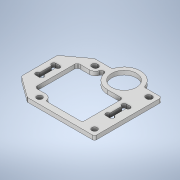
# Autodesk Inventor part: Trunk_chest_side_frame
Saved by Autodesk Inventor 2020.4 (Build 244396000, 396)
## iProperties
Created: 2021-09-08
Part Number: Trunk_chest_side_frame
Material: アルミニウム 2014-T4
Document SubType Name: Modeling
Designer: Masato Kubotera
Density: 2.8 g/cm^3
Appearance: 滑らか - 淡い灰色
Mass: 2.76884 g
Surface Area: 18.8552 cm^2
Volume: 0.988872 cm^3
Description: A2017 T2
Author: moonk
Autodesk Inventor part; units mm, degrees
ref_plane "YZ Plane" through (0, 0, 0) normal (1, 0, 0) x (0, 1, 0)
ref_plane "XZ Plane" through (0, 0, 0) normal (0, 1, 0) x (-1, 0, 0)
ref_plane "XY Plane" through (0, 0, 0) normal (0, 0, 1) x (1, 0, 0)
sketch "スケッチ1" plane through (0, 0, 0) normal (0, 0, 1) x (1, 0, 0)
  circle A0 centre (0, 0) radius 6.05
  arc A1 (2, -7.7976) -> (2, 7.7976) centre (0, 0) ccw
  line L0 (-31, 0) -> (0, 0) construction
  line L1 (-19.51, 24.01) -> (-9.49, 24.01)
  line L2 (-9.49, 24.01) -> (-9.49, 21.99)
  line L3 (-9.49, 21.99) -> (-19.51, 21.99)
  line L4 (-19.51, 21.99) -> (-19.51, 24.01)
  line L5 (-19.51, 24.01) -> (-9.49, 21.99) construction
  line L6 (-9.49, 24.01) -> (-19.51, 21.99) construction
  line L7 (-19.5, 24) -> (-9.5, 24) construction
  line L8 (-9.5, 24) -> (-9.5, 22) construction
  line L9 (-9.5, 22) -> (-19.5, 22) construction
  line L10 (-19.5, 22) -> (-19.5, 24) construction
  line L11 (-19.5, 24) -> (-9.5, 22) construction
  line L12 (-9.5, 24) -> (-19.5, 22) construction
  line L13 (-19.51, 23) -> (-9.49, 23) construction
  arc A2 (-17.41, 24.01) -> (-19.51, 24.01) centre (-18.46, 24.01) ccw
  arc A3 (-19.51, 21.99) -> (-17.41, 21.99) centre (-18.46, 21.99) ccw
  line L14 (-14.5, 24) -> (-14.5, 21.99) construction
  arc A4 (-9.49, 24.01) -> (-11.59, 24.01) centre (-10.54, 24.01) ccw
  arc A5 (-11.59, 21.99) -> (-9.49, 21.99) centre (-10.54, 21.99) ccw
  line L15 (-28, 13.5) -> (-1, 13.5) construction
  line L16 (-1, 13.5) -> (-1, -13.5) construction
  line L17 (-1, -13.5) -> (-28, -13.5) construction
  line L18 (-28, -13.5) -> (-28, 13.5) construction
  line L19 (-28, 13.5) -> (-1, -13.5) construction
  line L20 (-1, 13.5) -> (-28, -13.5) construction
  line L21 (-14.5, 13.5) -> (-14.5, -13.5) construction
  line L22 (-19.51, -10.49) -> (-9.49, -10.49)
  line L23 (-9.49, -10.49) -> (-9.49, -12.51)
  line L24 (-9.49, -12.51) -> (-19.51, -12.51)
  line L25 (-19.51, -12.51) -> (-19.51, -10.49)
  line L26 (-19.51, -10.49) -> (-9.49, -12.51) construction
  line L27 (-9.49, -10.49) -> (-19.51, -12.51) construction
  line L28 (-19.5, -10.5) -> (-9.5, -10.5) construction
  line L29 (-9.5, -10.5) -> (-9.5, -12.5) construction
  line L30 (-9.5, -12.5) -> (-19.5, -12.5) construction
  line L31 (-19.5, -12.5) -> (-19.5, -10.5) construction
  line L32 (-19.5, -10.5) -> (-9.5, -12.5) construction
  line L33 (-9.5, -10.5) -> (-19.5, -12.5) construction
  line L34 (-19.51, -11.5) -> (-9.49, -11.5) construction
  arc A6 (-17.41, -10.49) -> (-19.51, -10.49) centre (-18.46, -10.49) ccw
  arc A7 (-19.51, -12.51) -> (-17.41, -12.51) centre (-18.46, -12.51) ccw
  line L35 (-14.5, -10.5) -> (-14.5, -12.51) construction
  arc A8 (-9.49, -10.49) -> (-11.59, -10.49) centre (-10.54, -10.49) ccw
  arc A9 (-11.59, -12.51) -> (-9.49, -12.51) centre (-10.54, -12.51) ccw
  line L36 (-31, 16.5) -> (-31, -16.5)
  line L37 (-31, -16.5) -> (2, -16.5)
  line L38 (2, -16.5) -> (2, -7.7976)
  line L39 (2, 7.7976) -> (2, 16.5)
  arc A10 (-28, 10.5) -> (-25, 13.5) centre (-28, 13.5) ccw
  line L40 (-28, 10.5) -> (-28, -7.5)
  line L41 (-28, -7.5) -> (-8.05, -7.5)
  line L42 (-8.05, -7.5) -> (-8.05, 0)
  arc A11 (-1, 7.9876) -> (-8.05, 0) centre (0, 0) ccw
  line L43 (-1, 10) -> (-1, 7.9876)
  circle A12 centre (-28, 13.5) radius 1.35
  arc A13 (0.35, 13.5) -> (-2.35, 13.5) centre (-1, 13.5) ccw
  arc A14 (-2.35, 13) -> (0.35, 13) centre (-1, 13) ccw
  arc A15 (-4, 13) -> (-1, 10) centre (-1, 13) ccw
  line L44 (0.35, 13) -> (0.35, 13.5)
  line L45 (-2.35, 13.5) -> (-2.35, 13)
  arc A16 (-2.35, -13.5) -> (0.35, -13.5) centre (-1, -13.5) ccw
  arc A17 (0.35, -13) -> (-2.35, -13) centre (-1, -13) ccw
  line L46 (0.35, -13) -> (0.35, -13.5)
  line L47 (-2.35, -13.5) -> (-2.35, -13)
  circle A18 centre (-28, -13.5) radius 1.35
  line L48 (-3.555, 24) -> (-3.555, 22) construction
  line L49 (-25.555, 21.9799) -> (-25.555, 24) construction
  line L50 (-25.555, 24) -> (-3.555, 22) construction
  line L51 (-3.555, 24) -> (-25.555, 21.9799) construction
  line L52 (-23.377, 27) -> (-5.777, 27)
  line L53 (-24.242, 19) -> (-4.7733, 19)
  line L54 (-4, 13) -> (-4, 13.5)
  line L55 (-23.377, 27) -> (-31, 16.5)
  line L56 (-5.777, 27) -> (2, 16.5)
  line L57 (-31, 16.5) -> (2, 16.5) construction
  line L58 (-24.242, 19) -> (-25, 17.9559)
  line L59 (-25, 17.9559) -> (-25, 13.5)
  line L60 (-4.7733, 19) -> (-4, 17.9559)
  line L61 (-4, 17.9559) -> (-4, 13.5)
  line L62 (-25, 17.9559) -> (-4, 17.9559) construction
  point P0 (-14.5, 23)
  point P1 (-14.5, 0)
  point P2 (-14.5, -11.5)
  point P3 (-14.5, 22.995)
  point P4 (-11.59, -10.49)
  point P5 (-11.59, -12.51)
  point P6 (-17.41, -12.51)
  point P7 (-17.41, 21.99)
  dimension "d96" = 12.1
  dimension "d215" = 10
  dimension "d216" = 2
  dimension "d217" = 0.01
  dimension "d219" = 0.01
  dimension "d220" = 1.05
  dimension "d222" = 27
  dimension "d223" = 27
  dimension "d226" = 10
  dimension "d227" = 2
  dimension "d228" = 0.01
  dimension "d229" = 0.01
  dimension "d230" = 1.05
  dimension "d231" = 32.5
  dimension "d238" = 3
  dimension "d241" = 3
  dimension "d244" = 2
  dimension "d245" = 3
  dimension "d246" = 3
  dimension "d251" = 2
  dimension "d252" = 3
  dimension "d255" = 1
  dimension "d257" = 2.7
  dimension "d259" = 2.7
  dimension "d260" = 0.5
  dimension "d263" = 4
  dimension "d265" = 22
  dimension "d266" = 3
  dimension "d267" = 3
  dimension "d271" = 3
  dimension "d272" = 3
  dimension "d273" = 3
  dimension "d274" = 3
  dimension "d276" = 4
  constraints: 128 end point, 32 point on circle, 23 point on line, 22 midpoint, 19 centre point, 19 parallel, 19 symmetric about line, 9 perpendicular, 7 coincident, 7 horizontal, 5 vertical, 4 tangent, 1 collinear, 1 concentric, 11 other
  measures "d96" diameter of A0
  measures "d215" distance of L8.end L9.end
  measures "d216" distance of L7.end L8.end
  measures "d217" horizontal distance of L1.start L7.start
  measures "d219" horizontal distance of L7.start L1.start
  measures "d220" radius of A2
  measures "d222" distance of L16.end L17.end
  measures "d223" distance of L15.end L16.end
  measures "d226" distance of L30.start L31.start
  measures "d227" distance of L33.start L30.start
  measures "d228" horizontal distance of L25.end L31.end
  measures "d229" horizontal distance of L31.end L25.end
  measures "d230" radius of A6
  measures "d231" distance of L31.end L9.end
  measures "d238" vertical distance of L16.end L33.start
  measures "d241" horizontal distance of L17.end L36.end
  measures "d244" radial gap between concentric circles of A1 A0
  measures "d245" horizontal distance of L36.start L40.start
  measures "d246" horizontal distance of L39.start L43.start
  measures "d251" radial gap between concentric circles of A11 A0
  measures "d252" distance from line of L31.end L41
  measures "d255" distance from line of L16 point (0, 0)
  measures "d257" diameter of A12
  measures "d259" diameter of A13
  measures "d260" distance of A14.centre L15.end
  measures "d263" distance between parallel lines of L37 L30
  measures "d265" distance between parallel lines of L48 L49
  measures "d266" distance between parallel lines of L52 L7
  measures "d267" distance from line of L36.end L17
  measures "d271" distance between parallel lines of L53 L9
  measures "d272" radius of A10
  measures "d273" radius of A15
  measures "d274" horizontal distance of L36.start A10.centre
  measures "d276" distance between parallel lines of L55 L58
extrude "押し出し1" add sketch "スケッチ1" along normal blind 2
fillet "フィレット1" radius 1 9 edges at (-1, 7.9876, 1) (-8.05, -7.5, 1) (-28, -7.5, 1) (-28, 10.5, 1) (-1, 10, 1) (-25, 17.9559, 1) (-24.242, 19, 1) (-4.7733, 19, 1) (-4, 17.9559, 1)
fillet "フィレット2" radius 1 8 edges at (-31, -16.5, 1) (2, -7.7976, 1) (2, -16.5, 1) (2, 7.7976, 1) (-31, 16.5, 1) (-23.377, 27, 1) (-5.777, 27, 1) (2, 16.5, 1)
